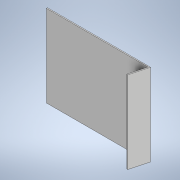
# Autodesk Inventor part: bottomCover
Saved by Autodesk Inventor 2020.3 (Build 243373000, 373)
## iProperties
Created: 2021-03-06
Part Number: bottomCover
Material: Generic
Document SubType Name: Modeling
Designer: allofus
Density: 1 g/cm^3
Appearance: Default
Author: allofus
Autodesk Inventor part; units mm, degrees
ref_plane "YZ Plane" through (0, 0, 0) normal (1, 0, 0) x (0, 1, 0)
ref_plane "XZ Plane" through (0, 0, 0) normal (0, 1, 0) x (-1, 0, 0)
ref_plane "XY Plane" through (0, 0, 0) normal (0, 0, 1) x (1, 0, 0)
sketch "Sketch1" plane through (0, 0, 0) normal (0, 1, 0) x (-1, 0, 0)
  line L0 (0, 0) -> (5, 0)
  line L1 (5, 161) -> (0, 161)
  line L2 (0, 0) -> (197, 0)
  line L3 (197, 0) -> (197, 2)
  line L4 (197, 2) -> (0, 2)
  line L5 (0, 2) -> (0, 0)
  line L6 (0, 2) -> (8.9293, 35.3244)
  line L7 (0, 2) -> (34.5, 2) construction
  line L8 (8.9293, 35.3244) -> (6.9974, 35.8421)
  line L9 (6.9974, 35.8421) -> (-2.6065, 0)
  line L10 (-2.6065, 0) -> (0, 0)
  line L11 (8.9293, 35.3244) -> (6.8587, 35.3244)
  dimension "d1" = 5
  dimension "d2" = 197
  dimension "d3" = 2
  dimension "d4" = 34.5
  dimension "d5" = 75
  dimension "d6" = 2
  constraints: 24 end point, 4 horizontal, 3 parallel, 3 perpendicular, 1 collinear, 1 equal length, 1 point on line
  measures "d1" distance of L1.start L1.end
  measures "d2" distance of L4.end L3.end
  measures "d3" distance of L3.end L2.end
  measures "d4" distance of L4.end L6.end
  measures "d5" angle of L7 L6
  measures "d6" distance of L6.end L8.end
extrude "Extrusion1" add sketch "Sketch1" along normal blind 161 contours L5 L4 L3 L2 L0 | L10 L9 L11 L6 L5
sketch "Sketch2" plane through (-197, 0, 2) normal (-1, 0, 0) x (0, 0, 1)
  line L0 (-2, 0) -> (0, 0) projected
  line L1 (0, 161) -> (33.3244, 161) projected
  line L2 (-2, 0) -> (0, 0)
  line L3 (0, 0) -> (0, 161)
  line L4 (0, 161) -> (-2, 161)
  line L5 (-2, 161) -> (-2, 0)
  constraints: 8 end point, 2 parallel, 1 horizontal, 1 perpendicular
extrude "Extrusion2" add sketch "Sketch2" along normal blind 3
body "Solid1"
